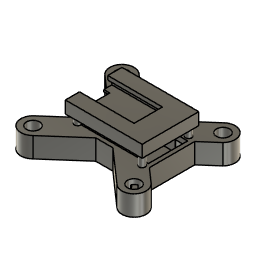
Drone V2 (Autodesk Fusion 360 design; units mm, degrees)
Autodesk Fusion 360 part; units mm, degrees
sketch "Skizze1" plane through (0, 0, 0) normal (0, 0, 1) x (1, 0, 0)
  line L0 (-50, 40) -> (0, 40) construction
  circle A0 centre (-50, 40) radius 3.25
  circle A1 centre (0, 40) radius 3.25
  line L1 (-25, 40) -> (-25, -4) construction
  line L2 (-25, -4) -> (0, -4) construction
  line L3 (0, -4) -> (-50, -4) construction
  circle A2 centre (-50, -4) radius 3.25
  circle A3 centre (0, -4) radius 3.25
  circle A4 centre (-50, 40) radius 6
  circle A5 centre (0, 40) radius 6
  circle A6 centre (0, -4) radius 6
  circle A7 centre (-50, -4) radius 6
  line L4 (-50, -4) -> (0, 40) construction
  line L5 (0, -4) -> (-50, 40) construction
  line L6 (-50, 40) -> (-50, 46) construction
  line L7 (-50, 40) -> (-49.8093, 40.2167) construction
  line L8 (-50, 40) -> (-45.7574, 44.2426) construction
  line L9 (-50, 40) -> (-44, 40) construction
  line L10 (-50, 40) -> (-56, 40) construction
  line L11 (-50, 40) -> (-54.2426, 35.7574) construction
  line L12 (0, -4) -> (6, -4) construction
  line L13 (0, -4) -> (4.2426, 0.2426) construction
  line L14 (0, -4) -> (6, -4) construction
  line L15 (0, -4) -> (0, -10) construction
  line L16 (0, -4) -> (-4.2426, -8.2426) construction
  line L17 (-4.2426, -8.2426) -> (-54.2426, 35.7574)
  line L18 (4.2426, 0.2426) -> (-45.7574, 44.2426)
  line L19 (0, 40) -> (0, 46) construction
  line L20 (0, 40) -> (-4.2426, 44.2426) construction
  line L21 (0, 40) -> (4.2426, 35.7574) construction
  line L22 (0, 40) -> (6, 40) construction
  line L23 (-50, -4) -> (-45.7574, -8.2426) construction
  line L24 (-50, -4) -> (-44, -4) construction
  line L25 (-50, -4) -> (-54.2426, 0.2426) construction
  line L26 (-50, -4) -> (-44, -4) construction
  line L27 (-54.2426, 0.2426) -> (-4.2426, 44.2426)
  line L28 (4.2426, 35.7574) -> (-45.7574, -8.2426)
  line L29 (-3.2166, 6.8068) -> (-3.2166, 29.1932)
  line L30 (-40.3073, 12.5057) -> (-40.3073, 23.4943)
  line L31 (-20.7574, 6.2903) -> (-29.2426, 6.2903)
  line L32 (-20.7574, 29.7097) -> (-29.2426, 29.7097)
  dimension "d2" = 6.5
  dimension "d3" = 6.5
  dimension "d4" = 6.5
  dimension "d5" = 6.5
  dimension "d6" = 12
  dimension "d7" = 12
  dimension "d8" = 12
  dimension "d9" = 45
  dimension "d10" = 135
  dimension "d11" = 6
  dimension "d12" = 45
  dimension "d13" = 135
  dimension "d14" = 135
  dimension "d15" = 45
  dimension "d16" = 6
  dimension "d17" = 45
  dimension "d18" = 135
  constraint horizontal L0
  constraint coincident L0.start A0.centre
  constraint coincident L0.end A1.centre
  constraint midpoint L0 L1.start
  constraint perpendicular L0 L1
  constraint perpendicular L1 L2
  constraint perpendicular L1 L3
  constraint coincident L3.end A2.centre
  constraint coincident L2.end L3.start
  constraint concentric A0 A4
  constraint concentric A1 A5
  constraint concentric A3 A6
  constraint concentric A2 A7
  constraint coincident A4 L6.end
  constraint vertical L6
  constraint perpendicular L5 L7
  constraint horizontal L9
  constraint coincident A4 L10.end
  constraint horizontal L10
  constraint coincident A6 L12.end
  constraint parallel L2 L12
  constraint horizontal L14
  constraint coincident A6 L15.end
  constraint vertical L15
  constraint coincident A5 L19.end
  constraint perpendicular L0 L19
  constraint horizontal L22
  constraint horizontal L24
  constraint horizontal L26
  constraint parallel L27 L28
  constraint coincident L18 L29.start
  constraint coincident L28 L29.end
  constraint vertical L29
  constraint coincident L27 L30.start
  constraint coincident L17 L30.end
  constraint parallel L29 L30
  constraint coincident L17 L31.start
  constraint coincident L28 L31.end
  constraint perpendicular L1 L31
  constraint coincident L27 L32.start
  constraint coincident L18 L32.end
  constraint perpendicular L1 L32
  measures "d2" diameter of A0
  measures "d3" diameter of A1
  measures "d4" diameter of A2
  measures "d5" diameter of A3
  measures "d6" diameter of A5
  measures "d7" diameter of A6
  measures "d8" diameter of A7
  measures "d9" angle of L8 L9
  measures "d10" angle of L10 L11
  measures "d11" distance of L2.end L13.end
  measures "d12" angle of L13 L14
  measures "d13" angle of L15 L16
  measures "d14" angle of L19 L20
  measures "d15" angle of L21 L22
  measures "d16" distance of L3.end L23.end
  measures "d17" angle of L23 L24
  measures "d18" angle of L25 L26
extrude "Extrusion1" add sketch "Skizze1" along normal blind 10 contours A4 L17 | A4 L17 L18 L27 | A5 L18 L27 L28 | L17 L18 L27 L28 | A7 L17 L27 L28 | A6 L17 L18 L28 | A5 L28 | A7 L27 | A6 L18 picked at (-55.035, 39.3919) picked at (-3.2811, 43.8676) picked at (-46.7227, -7.8704) picked at (-3.2811, -7.8676)
extrude "Extrusion2" add sketch "Skizze1" along normal blind 10 contours L18 L27 L32 | L17 L27 L30 | L18 L28 L29 | L17 L28 L31
sketch "Skizze2" plane through (0, 0, 10) normal (0, 0, 1) x (-1, 0, 0)
  circle A0 centre (0, -40) radius 3.25
  circle A1 centre (50, 4) radius 3.25
  circle A2 centre (50, -40) radius 3.25
  circle A3 centre (0, 4) radius 3.25
  line L0 (29.2426, -29.7097) -> (45.7574, -44.2426)
  arc A4 (45.7574, -44.2426) -> (54.2426, -35.7574) centre (50, -40) ccw
  line L1 (54.2426, -35.7574) -> (40.3073, -23.4943)
  line L2 (40.3073, -23.4943) -> (40.3073, -12.5057)
  line L3 (40.3073, -12.5057) -> (54.2426, -0.2426)
  arc A5 (54.2426, -0.2426) -> (45.7574, 8.2426) centre (50, 4) ccw
  line L4 (45.7574, 8.2426) -> (29.2426, -6.2903)
  line L5 (29.2426, -6.2903) -> (20.7574, -6.2903)
  line L6 (20.7574, -6.2903) -> (4.2426, 8.2426)
  arc A6 (4.2426, 8.2426) -> (-4.2426, -0.2426) centre (0, 4) ccw
  line L7 (-4.2426, -0.2426) -> (3.2166, -6.8068)
  line L8 (3.2166, -6.8068) -> (3.2166, -29.1932)
  line L9 (3.2166, -29.1932) -> (-4.2426, -35.7574)
  arc A7 (-4.2426, -35.7574) -> (4.2426, -44.2426) centre (0, -40) ccw
  line L10 (4.2426, -44.2426) -> (20.7574, -29.7097)
  line L11 (20.7574, -29.7097) -> (29.2426, -29.7097)
  line L12 (5.2166, -8.2903) -> (38.3073, -8.2903) construction
  line L13 (38.3073, -8.2903) -> (38.3073, -27.7097) construction
  line L14 (38.3073, -27.7097) -> (5.2166, -27.7097) construction
  line L15 (5.2166, -27.7097) -> (5.2166, -8.2903) construction
  line L16 (3.2166, -6.8068) -> (3.2166, -29.1932) construction
  line L17 (5.2166, -8.2903) -> (38.3073, -8.2903)
  line L18 (38.3073, -8.2903) -> (38.3073, -27.7097)
  line L19 (38.3073, -27.7097) -> (5.2166, -27.7097)
  line L20 (5.2166, -27.7097) -> (5.2166, -8.2903)
  dimension "d24" = 2
  dimension "d25" = 2
  dimension "d26" = 2
  dimension "d27" = 2
  constraint perpendicular L8 L12
  constraint perpendicular L12 L13
  constraint perpendicular L13 L14
  constraint horizontal L17
  constraint vertical L18
  constraint horizontal L19
  constraint vertical L20
  measures "d24" distance of L11 L14
  measures "d25" distance of L5 L12
  measures "d26" distance of L15 L16
  measures "d27" distance of L2 L13
extrude "Extrusion3" cut sketch "Skizze2" against normal blind 8 contours L17 L18 L19 L20
sketch "Skizze3" plane through (0, 0, 10) normal (0, 0, 1) x (-1, 0, 0)
  line L0 (38.3073, -8.2903) -> (38.3073, -27.7097)
  line L1 (38.3073, -27.7097) -> (5.2166, -27.7097)
  line L2 (5.2166, -27.7097) -> (5.2166, -8.2903)
  line L3 (5.2166, -8.2903) -> (38.3073, -8.2903)
  circle A0 centre (0, -40) radius 3.25
  circle A1 centre (50, 4) radius 3.25
  circle A2 centre (50, -40) radius 3.25
  circle A3 centre (0, 4) radius 3.25
  line L4 (29.2426, -29.7097) -> (45.7574, -44.2426)
  arc A4 (45.7574, -44.2426) -> (54.2426, -35.7574) centre (50, -40) ccw
  line L5 (54.2426, -35.7574) -> (40.3073, -23.4943)
  line L6 (40.3073, -23.4943) -> (40.3073, -12.5057)
  line L7 (40.3073, -12.5057) -> (54.2426, -0.2426)
  arc A5 (54.2426, -0.2426) -> (45.7574, 8.2426) centre (50, 4) ccw
  line L8 (45.7574, 8.2426) -> (29.2426, -6.2903)
  line L9 (29.2426, -6.2903) -> (20.7574, -6.2903)
  line L10 (20.7574, -6.2903) -> (4.2426, 8.2426)
  arc A6 (4.2426, 8.2426) -> (-4.2426, -0.2426) centre (0, 4) ccw
  line L11 (-4.2426, -0.2426) -> (3.2166, -6.8068)
  line L12 (3.2166, -6.8068) -> (3.2166, -29.1932)
  line L13 (3.2166, -29.1932) -> (-4.2426, -35.7574)
  arc A7 (-4.2426, -35.7574) -> (4.2426, -44.2426) centre (0, -40) ccw
  line L14 (4.2426, -44.2426) -> (20.7574, -29.7097)
  line L15 (20.7574, -29.7097) -> (29.2426, -29.7097)
  line L16 (48.8732, -36.9516) -> (38.0802, -26.1585)
  line L17 (48.8732, -36.9516) -> (64.1369, -36.9516) construction
  line L18 (46.8537, -39.1856) -> (34.6878, -27.7097)
  line L19 (48.8732, -36.9516) -> (46.8537, -39.1856)
  line L20 (38.0802, -26.1585) -> (34.6878, -27.7097)
  line L21 (1.4355, -37.0842) -> (7.4315, -27.7097)
  line L22 (11.379, -27.7097) -> (11.379, -27.9297)
  line L23 (11.379, -27.9297) -> (2.8213, -38.3867)
  line L24 (11.379, -27.7097) -> (7.4315, -27.7097)
  line L25 (2.8213, -38.3867) -> (1.4355, -37.0842)
  line L26 (1.0685, 0.9307) -> (9.1829, -8.2903)
  line L27 (2.9716, 2.684) -> (12.3168, -8.2903)
  line L28 (47.853, 1.5602) -> (47.9543, 1.6753)
  line L29 (47.9543, 1.6753) -> (38.3073, -9.8074)
  line L30 (46.9218, 5.0426) -> (46.0785, 2.5527)
  line L31 (46.0785, 2.5527) -> (36.9689, -8.2903)
  line L32 (38.3073, -9.8074) -> (36.9689, -8.2903)
  line L33 (46.9218, 5.0426) -> (46.9218, 4.5082)
  line L34 (46.9218, 4.5082) -> (47.853, 1.5602)
  line L35 (2.9716, 2.684) -> (1.0685, 0.9307)
  line L36 (12.3168, -8.2903) -> (9.1829, -8.2903)
  line L37 (9.1829, -8.2903) -> (12.3168, -8.2903)
  dimension "d30" = 135
  constraint horizontal L17
  constraint coincident A2 L16.start
  constraint coincident A2 L18.start
  constraint coincident L1 L18.end
  constraint coincident A0 L21.start
  constraint coincident L1 L21.end
  constraint coincident L1 L22.start
  constraint perpendicular L1 L22
  constraint coincident A0 L23.end
  constraint coincident A3 L26.start
  constraint coincident L3 L26.end
  constraint perpendicular L14 L26
  constraint coincident A3 L27.start
  constraint coincident L3 L27.end
  constraint coincident A1 L28.start
  constraint coincident A1.centre L28
  constraint perpendicular L10 L28
  constraint coincident L0 L29.end
  constraint coincident A1 L30.start
  constraint tangent A1 L30
  constraint coincident L3 L31.end
  constraint parallel L29 L31
  constraint vertical L33
  constraint parallel L3 L36
  measures "d30" angle of L16 L17
extrude "Extrusion4" cut sketch "Skizze3" against normal blind 6 contours L0 L3 A1 L29 L30 L31 | L0 L1 A2 L16 L18 | L3 A3 L26 L27 L36 L37 | L1 A0 L21 L22 L23 L24
extrude "Extrusion5" add sketch "Skizze3" against normal blind 2.5 contours L0 L3 A1 L29 L30 L31 | L0 L1 A2 L16 L18 | L3 A3 L26 L27 L36 L37 | L1 A0 L21 L22 L23 L24
sketch "Skizze4" plane through (0, 0, 10) normal (0, 0, 1) x (-1, 0, 0)
  circle A0 centre (39, -29.5) radius 1.5
  circle A1 centre (7, -30) radius 1.5
  circle A2 centre (40, -8) radius 1.5
  circle A3 centre (6, -6) radius 1.5
  dimension "d35" = 3
  dimension "d36" = 3
  dimension "d37" = 3
  dimension "d38" = 3
  measures "d35" diameter of A0
  measures "d36" diameter of A1
  measures "d37" diameter of A2
  measures "d38" diameter of A3
extrude "Extrusion6" add sketch "Skizze4" along normal blind 5
sketch "Skizze5" plane through (0, 0, 15) normal (0, 0, 1) x (-1, 0, 0)
  circle A0 centre (40, -8) radius 1.5
  line L0 (4, -4) -> (42, -4)
  line L1 (42, -4) -> (42, -32)
  line L2 (42, -32) -> (4, -32)
  line L3 (4, -32) -> (4, -4)
  constraint horizontal L0
  constraint vertical L1
  constraint horizontal L2
  constraint vertical L3
extrude "Extrusion7" add sketch "Skizze5" along normal blind 1 contours A0 | L0 L1 L2 L3
sketch "Skizze6" plane through (0, 0, 16) normal (0, 0, 1) x (-1, 0, 0)
  line L0 (4, -32) -> (42, -32)
  line L1 (42, -32) -> (42, -4)
  line L2 (42, -4) -> (4, -4)
  line L3 (4, -4) -> (4, -32)
  line L4 (42, -27) -> (10, -27)
  line L5 (10, -27) -> (10, -9)
  line L6 (10, -9) -> (42, -9)
  line L7 (42, -9) -> (42, -4)
  line L8 (4, -4) -> (4, -32)
  line L9 (42, -32) -> (42, -27)
  dimension "d43" = 5
  dimension "d44" = 5
  dimension "d45" = 6
  constraint horizontal L4
  constraint perpendicular L4 L5
  constraint coincident L1 L6.end
  constraint perpendicular L1 L6
  constraint coincident L1.end L2.start
  constraint coincident L2.end L3.start
  constraint coincident L0.start L3.end
  constraint coincident L0.end L1.start
  constraint perpendicular L4 L9
  measures "d43" distance of L0 L4
  measures "d44" distance of L2 L6
  measures "d45" distance of L5 L8
extrude "Extrusion8" add sketch "Skizze6" along normal blind 5 contours L0 L1 L2 L3 L4 L5 L6 L7 L8 L9
sketch "Skizze7" plane through (0, 0, 16) normal (0, 0, 1) x (-1, 0, 0)
  line L0 (42, -9) -> (10, -9)
  line L1 (10, -9) -> (10, -27)
  line L2 (10, -27) -> (42, -27)
  line L3 (42, -27) -> (42, -9)
  line L4 (42, -23) -> (39, -23)
  line L5 (39, -23) -> (39, -13)
  line L6 (39, -13) -> (42, -13)
  line L7 (42, -23) -> (42, -13)
  constraint coincident L3 L4.start
  constraint perpendicular L3 L4
  constraint perpendicular L4 L5
  constraint coincident L3 L6.end
  constraint perpendicular L3 L6
extrude "Extrusion9" cut sketch "Skizze7" against normal blind 1 contours L3 L4 L5 L6 L7
sketch "Skizze8" plane through (0, 27, 0) normal (0, -1, 0) x (1, 0, 0)
  line L0 (-42, 16) -> (-10, 16)
  line L1 (-10, 16) -> (-10, 21)
  line L2 (-10, 21) -> (-42, 21)
  line L3 (-42, 21) -> (-42, 16)
  line L4 (-42, 19) -> (-10, 19)
  constraint coincident L3 L4.start
  constraint perpendicular L3 L4
extrude "Extrusion10" add sketch "Skizze8" along normal blind 2 contours L1 L2 L3 L4
sketch "Skizze9" plane through (0, 9, 0) normal (0, 1, 0) x (-1, 0, 0)
  line L0 (10, 16) -> (42, 16)
  line L1 (42, 16) -> (42, 21)
  line L2 (42, 21) -> (10, 21)
  line L3 (10, 21) -> (10, 16)
  line L4 (10, 19) -> (42, 19)
  constraint coincident L3 L4.start
  constraint coincident L1 L4.end
  constraint perpendicular L1 L4
extrude "Extrusion11" add sketch "Skizze9" along normal blind 2 contours L1 L2 L3 L4
sketch "Skizze10" plane through (-10, 0, 0) normal (-1, 0, 0) x (0, -1, 0)
  line L0 (-11, 19) -> (-11, 21)
  line L1 (-11, 21) -> (-25, 21)
  line L2 (-25, 21) -> (-25, 19)
  line L3 (-25, 19) -> (-27, 19)
  line L4 (-27, 19) -> (-27, 16)
  line L5 (-27, 16) -> (-9, 16)
  line L6 (-9, 16) -> (-9, 19)
  line L7 (-9, 19) -> (-11, 19)
  line L8 (-25, 19) -> (-11, 19)
  constraint coincident L2.end L3.start
  constraint coincident L0.start L7.end
extrude "Extrusion12" add sketch "Skizze10" along normal blind 5 contours L0 L1 L2 L8
